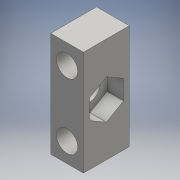
# Autodesk Inventor part: smallSprocketFixture
Saved by Autodesk Inventor 2016 (Build 200138000, 138)
## iProperties
Created: 2016-06-05
Part Number: smallSprocketFixture
Material: Generic
Document SubType Name: Modeling
Designer: hesaon
Density: 1 g/cm^3
Appearance: Default
Author: hesaon
Autodesk Inventor part; units mm, degrees
ref_plane "YZ Plane" through (0, 0, 0) normal (1, 0, 0) x (0, 1, 0)
ref_plane "XZ Plane" through (0, 0, 0) normal (0, 1, 0) x (-1, 0, 0)
ref_plane "XY Plane" through (0, 0, 0) normal (0, 0, 1) x (1, 0, 0)
sketch "Sketch1" plane through (0, 0, 0) normal (0, 1, 0) x (-1, 0, 0)
  line L0 (0, 0) -> (10, 0)
  line L1 (10, 0) -> (10, -32)
  line L2 (10, -32) -> (0, -32)
  line L3 (0, -32) -> (0, 0)
  circle A0 centre (5, -6) radius 3.25
  circle A1 centre (5, -26) radius 3.25
  dimension "t" = 10
  dimension "d2" = 6.5
  dimension "d3" = 6.5
  dimension "d4" = 6
  dimension "d5" = 6
  dimension "d6" = 5
  dimension "d7" = 5
  dimension "height" = 32
  constraints: 8 end point, 2 centre point, 2 parallel, 1 horizontal, 1 perpendicular
  measures "t" distance of L2.end L1.end
  measures "d2" diameter of A0
  measures "d3" diameter of A1
  measures "d4" distance from line of L0 A0.centre
  measures "d5" distance from line of L2 A1.centre
  measures "d6" distance from line of L3 A0.centre
  measures "d7" distance from line of L3 A1.centre
  measures "height" distance between parallel lines of L2 L0
extrude "Extrusion1" add sketch "Sketch1" along normal blind 14
sketch "Sketch2" plane through (0, 0, 0) normal (1, 0, 0) x (0, 0, -1)
  circle A0 centre (16, 7) radius 3.1
  line L0 (0, 0) -> (0, 14) projected
  line L1 (32, 0) -> (0, 0) projected
  dimension "d10" = 6.2
  dimension "d12" = 16
  dimension "d13" = 7
  constraints: 1 centre point
  measures "d10" diameter of A0
  measures "d12" distance from line of L0 A0.centre
  measures "d13" distance from line of L1 A0.centre
extrude "Extrusion2" cut sketch "Sketch2" against normal up to next
sketch "Sketch3" plane through (0, 0, 0) normal (1, 0, 0) x (0, 0, -1)
  circle A0 centre (16, 7) radius 3.1 projected
  line L0 (22.0044, 7) -> (19.0022, 1.8)
  line L1 (19.0022, 1.8) -> (12.9978, 1.8)
  line L2 (12.9978, 1.8) -> (9.9956, 7)
  line L3 (9.9956, 7) -> (12.9978, 12.2)
  line L4 (12.9978, 12.2) -> (19.0022, 12.2)
  line L5 (19.0022, 12.2) -> (22.0044, 7)
  line L6 (0, 14) -> (32, 14) projected
  point P0 (0, 0)
  point P1 (16, 12.2)
  dimension "d16" = 10.4
  constraints: 12 end point, 1 coincident, 1 midpoint, 1 parallel, 13 other
  measures "d16" distance between parallel lines of L1 L4
extrude "Extrusion3" cut sketch "Sketch3" against normal blind 5
equation "\"d6\" = 0.5 * t"
equation "\"d7\" = 0.5 * t"
equation "\"d12\" = 0.5 * height"
body "Solid1"
